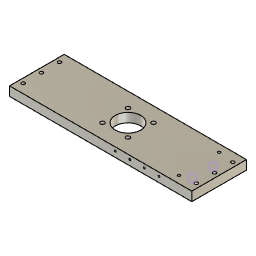
securing_structure_lid v106 (Autodesk Fusion 360 design; units mm, degrees)
Autodesk Fusion 360 part; units mm, degrees
note: some values were not read from the file. Chosen so that the rebuilt part matches the saved one: which face or edge a step refers to; how an offset face is resized; which pieces of a blend or face edit are solid. Set by a fixed rule: which sketch regions a step uses.
(part 1 of 2)
sketch "Sketch1" plane through (0, 0, 0) normal (0, 0, 1) x (1, 0, 0)
  line L0 (0, 0) -> (215, 0)
  line L1 (215, 0) -> (215, 55)
  line L2 (215, 55) -> (0, 55)
  line L3 (0, 55) -> (0, 0)
  line L4 (215, 55) -> (-215, 55)
  line L5 (-215, 55) -> (-215, -55)
  line L6 (-215, -55) -> (215, -55)
  line L7 (215, -55) -> (215, 55)
  dimension "d1" = 215
  dimension "d2" = 55
  dimension "d3" = 430
  dimension "d4" = 110
  constraint horizontal L0
  constraint vertical L1
  constraint horizontal L2
  constraint vertical L3
  constraint horizontal L4
  constraint vertical L5
  constraint horizontal L6
  constraint vertical L7
  measures "d1" distance of L0.start L0.end
  measures "d2" distance of L0.start L2.end
  measures "d3" distance of L1.end L4.end
  measures "d4" distance of L1.end L6.end
extrude "Extrude1" add sketch "Sketch1" along normal blind 170
sketch "Sketch2" plane through (0, 0, 0) normal (0, 0, 1) x (1, 0, 0)
  line L0 (0, 0) -> (-235, 0)
  line L1 (0, 0) -> (235, 0)
  line L2 (-235, 0) -> (235, 0)
  line L3 (235, 0) -> (235, 75)
  line L4 (235, 75) -> (-235, 75)
  line L5 (-235, 75) -> (-235, 0)
  line L6 (-235, 75) -> (235.5022, 75)
  line L7 (235.5022, 75) -> (235.5022, -75)
  line L8 (235.5022, -75) -> (-235, -75)
  line L9 (-235, -75) -> (-235, 75)
  line L10 (0, 0) -> (-215, 0)
  line L11 (-215, 0) -> (-215, 55)
  line L12 (-215, 55) -> (0, 55)
  line L13 (0, 55) -> (0, 0)
  line L14 (-215, 55) -> (215, 55)
  line L15 (215, 55) -> (215, -55)
  line L16 (215, -55) -> (-215, -55)
  line L17 (-215, -55) -> (-215, 55)
  dimension "d7" = 235
  dimension "d8" = 235
  dimension "d9" = 470
  dimension "d10" = 75
  dimension "d11" = 150
  dimension "d12" = 215
  dimension "d13" = 55
  dimension "d14" = 430
  dimension "d15" = 110
  constraint coincident L0.start L1.start
  constraint horizontal L0
  constraint parallel L0 L1
  constraint horizontal L2
  constraint vertical L3
  constraint horizontal L4
  constraint vertical L5
  constraint horizontal L6
  constraint vertical L7
  constraint horizontal L8
  constraint vertical L9
  constraint horizontal L10
  constraint vertical L11
  constraint horizontal L12
  constraint vertical L13
  constraint horizontal L14
  constraint vertical L15
  constraint horizontal L16
  constraint vertical L17
  measures "d7" distance of L0.start L0.end
  measures "d8" distance of L0.start L1.end
  measures "d9" distance of L0.end L1.end
  measures "d10" distance of L0.end L4.end
  measures "d11" distance of L4.end L8.end
  measures "d12" distance of L0.start L10.end
  measures "d13" distance of L0.start L12.end
  measures "d14" distance of L11.end L14.end
  measures "d15" distance of L11.end L16.end
extrude "Extrude2" add sketch "Sketch2" along normal blind 190 contours L0 L1 L2 L3 L6 L7 L8 L9 L15 L16 L17 | L0 L1 L2 L3 L4 L5 L6 L9 L11 L12 L14 L15 L17
extrude "Extrude3" add 1 faces at (-71.6667, 18.3333, 170) along direction (0, 0, 1) blind 20
sketch "Sketch3" plane through (0, 0, 0) normal (0, 0, -1) x (1, 0, 0)
  line L0 (235.5022, 75) -> (-235, 75)
  line L1 (-235, 75) -> (-235, -75)
  line L2 (-235, -75) -> (235.5022, -75)
  line L3 (235.5022, -75) -> (235.5022, 75)
  line L4 (0, 0) -> (-215, 0)
  line L5 (-215, 0) -> (-215, 55)
  line L6 (-215, 55) -> (0, 55)
  line L7 (0, 55) -> (0, 0)
  line L8 (-215, 55) -> (215, 55)
  line L9 (215, 55) -> (215, -55)
  line L10 (215, -55) -> (-215, -55)
  line L11 (-215, -55) -> (-215, 55)
  dimension "d20" = 215
  dimension "d21" = 55
  dimension "d22" = 430
  dimension "d23" = 110
  constraint horizontal L4
  constraint vertical L5
  constraint horizontal L6
  constraint vertical L7
  constraint coincident L4.start L7.end
  constraint horizontal L8
  constraint vertical L9
  constraint horizontal L10
  constraint vertical L11
  measures "d20" distance of L4.start L4.end
  measures "d21" distance of L4.start L6.end
  measures "d22" distance of L5.end L8.end
  measures "d23" distance of L5.end L10.end
extrude "Extrude4" cut sketch "Sketch3" against normal blind 170 contours L4 L7 L8 L9 L10 L11 | L4 L5 L6 L7 L8 L11
sketch "Sketch4" plane through (0, -75, 0) normal (0, -1, 0) x (1, 0, 0)
  line L0 (-235, 0) -> (235.5022, 0)
  line L1 (235.5022, 0) -> (235.5022, 190)
  line L2 (235.5022, 190) -> (-235, 190)
  line L3 (-235, 190) -> (-235, 0)
  line L4 (0, 0) -> (-215, 0)
  line L5 (-215, 0) -> (-215, 170)
  line L6 (-215, 170) -> (0, 170)
  line L7 (0, 170) -> (0, 0)
  line L8 (0, 0) -> (215, 0)
  line L9 (215, 0) -> (215, 170)
  line L10 (215, 170) -> (0, 170)
  line L11 (0, 170) -> (0, 0)
  dimension "d26" = 215
  dimension "d27" = 170
  dimension "d28" = 215
  constraint horizontal L4
  constraint vertical L5
  constraint horizontal L6
  constraint vertical L7
  constraint coincident L4.start L7.end
  constraint horizontal L8
  constraint vertical L9
  constraint horizontal L10
  constraint vertical L11
  measures "d26" distance of L4.start L4.end
  measures "d27" distance of L4.start L6.end
  measures "d28" distance of L4.start L8.end
extrude "Extrude5" cut sketch "Sketch4" against normal blind 200 contours L0 L4 L5 L6 L7 L11 | L0 L7 L8 L9 L10 L11
sketch "Sketch5" plane through (0, 0, 190) normal (0, 0, 1) x (-1, 0, 0)
  line L0 (235, 75) -> (-235.5022, 75)
  line L1 (-235.5022, 75) -> (-235.5022, -75)
  line L2 (-235.5022, -75) -> (235, -75)
  line L3 (235, -75) -> (235, 75)
  circle A0 centre (0, 0) radius 17.4
  dimension "d31" = 34.8
  constraint coincident A0.centre origin
  measures "d31" diameter of A0
extrude "Extrude6" cut sketch "Sketch5" against normal blind 60 contours A0
extrude "Extrude7" add 1 faces at (-235, 25, 63.3333) along direction (-1, 0, 0) blind 5
extrude "Extrude8" add 1 faces at (235.5022, 25, 63.3333) along direction (1, 0, 0) blind 5
extrude "Extrude9" cut 1 faces at (-215, -25, 56.6667) along direction (-1, 0, 0) blind 5
extrude "Extrude10" cut 1 faces at (215, -25, 56.6667) along direction (1, 0, 0) blind 5
extrude "Extrude11" add 1 faces at (-240, 25, 63.3333) along direction (-1, 0, 0) blind 5
extrude "Extrude12" cut 1 faces at (220, -25, 56.6667) along direction (1, 0, 0) blind 5
extrude "Extrude13" cut 1 faces at (-220, -25, 56.6667) along direction (-1, 0, 0) blind 5
extrude "Extrude14" add 1 faces at (240.5022, 25, 63.3333) along direction (1, 0, 0) blind 5
extrude "Extrude15" add 2 faces at (-231.6667, -25, 0) (238.6682, -25, 0) along direction (0, 0, -1) blind 0.719
sketch "Sketch6" plane through (-245, 0, 0) normal (-1, 0, 0) x (0, -1, 0)
  line L0 (75, -0.719) -> (75, 190)
  line L1 (75, 190) -> (-75, 190)
  line L2 (-75, 190) -> (-75, -0.719)
  line L3 (-75, -0.719) -> (75, -0.719)
  line L4 (-75, -0.719) -> (75, -0.719)
  line L5 (75, -0.719) -> (75, 19.281)
  line L6 (75, 19.281) -> (-75, 19.281)
  line L7 (-75, 19.281) -> (-75, -0.719)
  dimension "d52" = 20
  constraint horizontal L4
  constraint vertical L5
  constraint horizontal L6
  constraint vertical L7
  constraint coincident L0 L5.end
  constraint coincident L2.end L3.start
  measures "d52" distance of L2.end L6.end
extrude "Extrude16" add sketch "Sketch6" along normal blind 40 contours L0 L2 L3 L4 L5 L6 L7
sketch "Sketch7" plane through (245.5022, 0, 0) normal (1, 0, 0) x (0, 1, 0)
  line L0 (75, -0.719) -> (75, 190)
  line L1 (75, 190) -> (-75, 190)
  line L2 (-75, 190) -> (-75, -0.719)
  line L3 (-75, -0.719) -> (75, -0.719)
  line L4 (-75, -0.719) -> (75, -0.719)
  line L5 (75, -0.719) -> (75, 19.281)
  line L6 (75, 19.281) -> (-75, 19.281)
  line L7 (-75, 19.281) -> (-75, -0.719)
  dimension "d55" = 20
  constraint horizontal L4
  constraint vertical L5
  constraint horizontal L6
  constraint vertical L7
  constraint coincident L0 L5.end
  constraint coincident L2.end L3.start
  measures "d55" distance of L2.end L6.end
extrude "Extrude17" add sketch "Sketch7" along normal blind 40 contours L0 L2 L3 L4 L5 L6 L7
sketch "Sketch8" plane through (0, 0, 19.281) normal (0, 0, 1) x (-1, 0, 0)
  line L0 (-245.5022, -75) -> (-245.5022, 75)
  line L1 (-245.5022, 75) -> (-285.5022, 75)
  line L2 (-285.5022, 75) -> (-285.5022, -75)
  line L3 (-285.5022, -75) -> (-245.5022, -75)
  line L4 (-285.5022, 0) -> (-245.5022, 0)
  line L5 (-265.5022, 0) -> (-265.5022, -50)
  line L6 (-265.5022, 0) -> (-265.5022, 50)
  line L7 (-265.5022, 50) -> (264.4978, 50)
  line L8 (264.4978, 50) -> (264.4978, -50)
  line L9 (264.4978, -50) -> (-265.5022, -50)
  line L10 (-265.5022, -50) -> (-265.5022, 50)
  dimension "d58" = 50
  dimension "d59" = 50
  dimension "d60" = 530
  dimension "d61" = 100
  constraint midpoint L2 L4.start
  constraint midpoint L0 L4.end
  constraint midpoint L4 L5.start
  constraint perpendicular L3 L5
  constraint perpendicular L4 L6
  constraint horizontal L7
  constraint vertical L8
  constraint horizontal L9
  constraint vertical L10
  measures "d58" distance of L5.start L5.end
  measures "d59" distance of L5.start L6.end
  measures "d60" distance of L6.end L7.end
  measures "d61" distance of L6.end L5.end
hole "Hole1" at (265.5022, 50, 19.281) at (265.5022, -50, 19.281) at (-264.4978, -50, 19.281) at (-264.4978, 50, 19.281) direction (0, 0, -1) diameter 7.035 depth 20 tip angle 180
thread "Thread1" "ISO Metric profile 8.0 M8x1 6H"
sketch "Sketch9" plane through (0, 0, 190) normal (0, 0, 1) x (-1, 0, 0)
  circle A0 centre (0, 0) radius 17.4
  line L0 (245, 75) -> (-245.5022, 75)
  line L1 (-245.5022, 75) -> (-245.5022, -75)
  line L2 (-245.5022, -75) -> (245, -75)
  line L3 (245, -75) -> (245, 75)
  line L4 (0, 0) -> (-35, 0)
  line L5 (-35, 0) -> (-35, -35)
  line L6 (-35, -35) -> (0, -35)
  line L7 (0, -35) -> (0, 0)
  line L8 (-35, -35) -> (35, -35)
  line L9 (35, -35) -> (35, 35)
  line L10 (35, 35) -> (-35, 35)
  line L11 (-35, 35) -> (-35, -35)
  dimension "d65" = 35
  dimension "d66" = 35
  dimension "d67" = 70
  dimension "d68" = 70
  constraint horizontal L4
  constraint vertical L5
  constraint horizontal L6
  constraint vertical L7
  constraint coincident A0.centre L4.start
  constraint horizontal L8
  constraint vertical L9
  constraint horizontal L10
  constraint vertical L11
  measures "d65" distance of A0.centre L4.end
  measures "d66" distance of A0.centre L6.end
  measures "d67" distance of L5.end L8.end
  measures "d68" distance of L5.end L10.end
hole "Hole2" at (-35, 35, 190) at (35, 35, 190) at (35, -35, 190) at (-35, -35, 190) direction (0, 0, -1) diameter 7.035 depth 10 tip angle 180
thread "Thread2" "ISO Metric profile 8.0 M8x1 6H"
sketch "Sketch10" plane through (0, 0, 190) normal (0, 0, 1) x (-1, 0, 0)
  circle A0 centre (-35, 35) radius 3.5175
  circle A1 centre (35, -35) radius 3.5175
  circle A2 centre (-35, -35) radius 3.5175
  circle A3 centre (35, 35) radius 3.5175
  circle A4 centre (0, 0) radius 17.4
  line L0 (245, 75) -> (-245.5022, 75)
  line L1 (-245.5022, 75) -> (-245.5022, -75)
  line L2 (-245.5022, -75) -> (245, -75)
  line L3 (245, -75) -> (245, 75)
  circle A5 centre (0, 0) radius 15
  dimension "d72" = 30
  constraint coincident A4.centre A5.centre
  measures "d72" diameter of A5
extrude "Extrude18" add sketch "Sketch10" against normal blind 20 contours A4
delete_face "DeleteFace1" 4 faces at (35.1753, 31.4869, 186.6667) (35.1753, -38.5131, 186.6667) (-34.8247, 31.4869, 186.6667) (-34.8247, -38.5131, 186.6667)
sketch "Sketch11" plane through (0, 0, 190) normal (0, 0, 1) x (-1, 0, 0)
  circle A0 centre (0, 0) radius 15
  line L0 (245, 75) -> (-245.5022, 75)
  line L1 (-245.5022, 75) -> (-245.5022, -75)
  line L2 (-245.5022, -75) -> (245, -75)
  line L3 (245, -75) -> (245, 75)
  line L4 (0, 0) -> (35, 0)
  line L5 (35, 0) -> (35, -35)
  line L6 (35, -35) -> (0, -35)
  line L7 (0, -35) -> (0, 0)
  line L8 (35, -35) -> (-35, -35)
  line L9 (-35, -35) -> (-35, 35)
  line L10 (-35, 35) -> (35, 35)
  line L11 (35, 35) -> (35, -35)
  constraint horizontal L4
  constraint vertical L5
  constraint horizontal L6
  constraint vertical L7
  constraint coincident A0.centre L4.start
  constraint horizontal L8
  constraint vertical L9
  constraint horizontal L10
  constraint vertical L11
hole "Hole3" at (-35, 35, 190) at (35, 35, 190) at (35, -35, 190) at (-35, -35, 190) direction (0, 0, -1) diameter 6.78 depth 10 tip angle 180
thread "Thread3" "ISO Metric profile 8.0 M8x1 6H" major diameter 8.147 minor diameter 7.035 pitch 1 angle 60 resizes the face on face at (-34.831, 31.6142, 186.6667) on face at (35.169, 31.6142, 186.6667) on face at (35.169, -38.3858, 186.6667) on face at (-34.831, -38.3858, 186.6667)
extrude "Extrude19" add 1 faces at (155, 0, 170) along direction (0, 0, -1) blind 38
extrude "Extrude20" cut 1 faces at (176.4014, -11.1796, 190) along direction (0, 0, -1) blind 38
hole "Hole4" at (35, -35, 180) direction (0, 0, -1) diameter 7.035 depth 38 tip angle 180
thread "Thread4" "ISO Metric profile 8.0 M8x1 6H"
sketch "Sketch12" plane through (0, 0, 180) normal (0, 0, 1) x (-1, 0, 0)
  circle A0 centre (35, -35) radius 3.5175
hole "Hole5" at (-35, 35, 180) direction (0, 0, -1) diameter 7.035 depth 38 tip angle 180
thread "Thread5" "ISO Metric profile 8.0 M8x1 6H"
sketch "Sketch13" plane through (0, 0, 180) normal (0, 0, 1) x (-1, 0, 0)
  circle A0 centre (-35, -35) radius 3.5175
hole "Hole6" at (35, 35, 180) direction (0, 0, -1) diameter 7.035 depth 38 tip angle 180
thread "Thread6" "ISO Metric profile 8.0 M8x1 6H"
sketch "Sketch14" plane through (0, 0, 180) normal (0, 0, 1) x (-1, 0, 0)
  circle A0 centre (35, 35) radius 3.5175
hole "Hole7" at (-35, -35, 180) direction (0, 0, -1) diameter 7.035 depth 38 tip angle 180
thread "Thread7" "ISO Metric profile 8.0 M8x1 6H"
sketch "Sketch15" plane through (285.5022, 0, 0) normal (1, 0, 0) x (0, 1, 0)
  line L0 (-75, 19.281) -> (-75, -0.719)
  line L1 (-75, -0.719) -> (75, -0.719)
  line L2 (75, -0.719) -> (75, 19.281)
  line L3 (75, 19.281) -> (-75, 19.281)
  line L4 (0, -0.719) -> (0, 9.281)
  dimension "d106" = 10
  constraint midpoint L1 L4.start
  constraint perpendicular L1 L4
  measures "d106" distance of L4.start L4.end
hole "Hole8" at (285.5022, 0, 9.281) direction (-1, 0, 0) diameter 7.035 depth 20 tip angle 180
thread "Thread8" "ISO Metric profile 8.0 M8x1 6H"
delete_face "DeleteFace2" 1 faces at (-265.7008, 53.3054, 12.6143)
delete_face "DeleteFace3" 1 faces at (-265.7008, -46.6946, 12.6143)
sketch "Sketch16" plane through (0, 0, 19.281) normal (0, 0, 1) x (-1, 0, 0)
  line L0 (245, 75) -> (245, -75)
  line L1 (245, -75) -> (285, -75)
  line L2 (285, -75) -> (285, 75)
  line L3 (285, 75) -> (245, 75)
  line L4 (285, -75) -> (265, -75)
  line L5 (265, -75) -> (265, -50)
  line L6 (265, -50) -> (285, -50)
  line L7 (285, -50) -> (285, -75)
  line L8 (285, 75) -> (265, 75)
  line L9 (265, 75) -> (265, 50)
  line L10 (265, 50) -> (285, 50)
  line L11 (285, 50) -> (285, 75)
  dimension "d110" = 20
  dimension "d111" = 25
  dimension "d112" = 20
  dimension "d113" = 25
  constraint horizontal L4
  constraint vertical L5
  constraint horizontal L6
  constraint vertical L7
  constraint coincident L1.end L2.start
  constraint horizontal L8
  constraint vertical L9
  constraint horizontal L10
  constraint vertical L11
  constraint coincident L2.end L3.start
  measures "d110" distance of L1.end L4.end
  measures "d111" distance of L1.end L6.end
  measures "d112" distance of L2.end L8.end
  measures "d113" distance of L2.end L10.end
hole "Hole9" at (-265, 50, 19.281) at (-265, -50, 19.281) direction (0, 0, -1) diameter 7.035 depth 20 tip angle 180
thread "Thread9" "ISO Metric profile 8.0 M8x1 6H"
sketch "Sketch17" plane through (0, 0, 152) normal (0, 0, 1) x (-1, 0, 0)
  circle A0 centre (-35, 35) radius 3.5175
  circle A1 centre (35, -35) radius 3.5175
  circle A2 centre (-35, -35) radius 3.5175
  circle A3 centre (35, 35) radius 3.5175
  circle A4 centre (0, 0) radius 15
  line L0 (245, 75) -> (-245.5022, 75)
  line L1 (-245.5022, 75) -> (-245.5022, -75)
  line L2 (-245.5022, -75) -> (245, -75)
  line L3 (245, -75) -> (245, 75)
  line L4 (-245.5022, 0) -> (-225.5022, 0)
  dimension "d117" = 20
  constraint midpoint L1 L4.start
  constraint perpendicular L1 L4
  measures "d117" distance of L4.start L4.end
hole "Hole10" at (225.5022, 0, 152) direction (0, 0, -1) diameter 7.035 depth 10 tip angle 180
thread "Thread10" "ISO Metric profile 8.0 M8x1 6H"
extrude "Extrude21" cut 1 faces at (225, -25, 43.5207) along direction (1, 0, 0) blind 0.5
delete_face "DeleteFace4" 1 faces at (264.2992, 53.3054, 12.6143)
delete_face "DeleteFace5" 1 faces at (264.2992, -46.6946, 12.6143)
delete_face "DeleteFace6" 1 faces at (-267.6374, -52.3275, 12.6143)
delete_face "DeleteFace7" 1 faces at (-267.6374, 47.6725, 12.6143)
extrude "Extrude22" cut 1 faces at (-285, -25, 5.9477) along direction (1, 0, 0) blind 40
extrude "Extrude23" cut 1 faces at (285.5022, 51.1692, 9.3686) along direction (-1, 0, 0) blind 40
extrude "Extrude24" cut 1 faces at (265.5022, 0.8784, 8.804) along direction (-1, 0, 0) blind 20
sketch "Sketch18" plane through (0, 0, -0.719) normal (0, 0, -1) x (1, 0, 0)
  line L0 (245.5022, -75) -> (245.5022, 75)
  line L1 (245.5022, 75) -> (225.5, 75)
  line L2 (225.5, 75) -> (225.5, -75)
  line L3 (225.5, -75) -> (245.5022, -75)
  line L4 (235.5011, -75) -> (235.5011, -50)
  line L5 (235.5011, 75) -> (235.5011, 50)
  line L6 (235.5011, -50) -> (235.5011, 0)
  line L7 (-235, -75) -> (-235, -50)
  line L8 (-235, 75) -> (-235, 50)
  line L9 (-235, 50) -> (-235, 0)
  dimension "d129" = 25
  dimension "d130" = 25
  dimension "d131" = 25
  dimension "d132" = 25
  constraint midpoint L3 L4.start
  constraint perpendicular L3 L4
  constraint midpoint L1 L5.start
  constraint perpendicular L1 L5
  constraint parallel L4 L6
  constraint parallel L6 L7
  constraint vertical L8
  constraint parallel L8 L9
  measures "d129" distance of L4.start L4.end
  measures "d130" distance of L5.start L5.end
  measures "d131" distance of L7.start L7.end
  measures "d132" distance of L8.start L8.end
hole "Hole11" at (-235, -50, -0.719) at (-235, 0, -0.719) at (-235, 50, -0.719) at (235.5011, 0, -0.719) at (235.5011, -50, -0.719) at (235.5011, 50, -0.719) direction (0, 0, 1) diameter 7.035 depth 20 tip angle 180
thread "Thread11" "ISO Metric profile 8.0 M8x1 6H"
delete_face "DeleteFace8" 1 faces at (225.6776, -3.5131, 148.6667)
sketch "Sketch19" plane through (0, 0, 152) normal (0, 0, 1) x (-1, 0, 0)
  circle A0 centre (-35, 35) radius 3.5175
  circle A1 centre (35, -35) radius 3.5175
  circle A2 centre (-35, -35) radius 3.5175
  circle A3 centre (35, 35) radius 3.5175
  circle A4 centre (0, 0) radius 15
  line L0 (245, 75) -> (-245.5022, 75)
  line L1 (-245.5022, 75) -> (-245.5022, -75)
  line L2 (-245.5022, -75) -> (245, -75)
  line L3 (245, -75) -> (245, 75)
  line L4 (-245.5022, 0) -> (-245, 0)
  line L5 (-245, 0) -> (-225, 0)
  line L6 (-225, 0) -> (-225, -13.746)
  line L7 (-225, -13.746) -> (-225, 13.746)
  dimension "d136" = 20
  dimension "d137" = 13.746
  dimension "d138" = 27.492
  constraint midpoint L1 L4.start
  constraint perpendicular L1 L4
  constraint perpendicular L1 L5
  constraint perpendicular L5 L6
  constraint perpendicular L5 L7
  measures "d136" distance of L4.end L5.end
  measures "d137" distance of L5.end L6.end
  measures "d138" distance of L6.end L7.end
hole "Hole12" at (225, 13.746, 152) at (225, -13.746, 152) direction (0, 0, -1) diameter 3.529 depth 10 tip angle 180
thread "Thread12" "ISO Metric profile 4.0 M4x0.5 6H"
sketch "Sketch20" plane through (0, 0, 152) normal (0, 0, 1) x (-1, 0, 0)
  circle A0 centre (-225, -13.746) radius 1.7644
  circle A1 centre (-225, 13.746) radius 1.7644
  circle A2 centre (-35, 35) radius 3.5175
  circle A3 centre (35, -35) radius 3.5175
  circle A4 centre (-35, -35) radius 3.5175
  circle A5 centre (35, 35) radius 3.5175
  circle A6 centre (0, 0) radius 15
  line L0 (245, 75) -> (-245.5022, 75)
  line L1 (-245.5022, 75) -> (-245.5022, -75)
  line L2 (-245.5022, -75) -> (245, -75)
  line L3 (245, -75) -> (245, 75)
  line L4 (-225, -13.746) -> (-215, -13.746)
  line L5 (-215, -13.746) -> (-215, 13.746)
  dimension "d142" = 10
  constraint coincident A0.centre L4.start
  constraint horizontal L4
  constraint perpendicular L4 L5
  measures "d142" distance of A0.centre L4.end
hole "Hole13" at (215, 13.746, 152) at (215, -13.746, 152) direction (0, 0, -1) diameter 3.529 depth 10 tip angle 180
thread "Thread13" "ISO Metric profile 4.0 M4x0.5 6H"
delete_face "DeleteFace9" 1 faces at (225.9201, 15.2516, 148.6667)
delete_face "DeleteFace10" 1 faces at (225.9201, -12.2404, 148.6667)
sketch "Sketch21" plane through (245.5022, 0, 0) normal (1, 0, 0) x (0, 1, 0)
  line L0 (75, 152) -> (-75, 152)
  line L1 (-75, 152) -> (-75, -0.719)
  line L2 (-75, -0.719) -> (75, -0.719)
  line L3 (75, -0.719) -> (75, 152)
  line L4 (0, 152) -> (-28.5, 152)
  line L5 (-28.5, 152) -> (-28.5, 142)
  line L6 (-28.5, 142) -> (0, 142)
  line L7 (0, 142) -> (0, 152)
  line L8 (-28.5, 152) -> (28.5, 152)
  line L9 (28.5, 152) -> (28.5, 142)
  line L10 (28.5, 142) -> (-28.5, 142)
  line L11 (-28.5, 142) -> (-28.5, 152)
  dimension "d146" = 28.5
  dimension "d147" = 10
  dimension "d148" = 57
  dimension "d149" = 10
  constraint horizontal L4
  constraint vertical L5
  constraint horizontal L6
  constraint vertical L7
  constraint midpoint L0 L4.start
  constraint horizontal L8
  constraint vertical L9
  constraint horizontal L10
  constraint vertical L11
  measures "d146" distance of L4.start L4.end
  measures "d147" distance of L4.start L6.end
  measures "d148" distance of L4.end L8.end
  measures "d149" distance of L4.end L5.end
extrude "Extrude25" cut sketch "Sketch21" against normal blind 10 contours L0 L7 L8 L9 L10 | L0 L4 L5 L6 L7 L8 L10 L11
sketch "Sketch22" plane through (235.5022, 0, 0) normal (1, 0, 0) x (0, 1, 0)
  line L0 (-28.5, 142) -> (28.5, 142)
  line L1 (28.5, 142) -> (28.5, 152)
  line L2 (28.5, 152) -> (-28.5, 152)
  line L3 (-28.5, 152) -> (-28.5, 142)
  line L4 (0, 142) -> (0, 147)
  dimension "d152" = 5
  constraint midpoint L0 L4.start
  constraint perpendicular L0 L4
  measures "d152" distance of L4.start L4.end
hole "Hole14" at (235.5022, 0, 147) direction (-1, 0, 0) diameter 6.78 depth 10 tip angle 180
thread "Thread14" "ISO Metric profile 8.0 M8x1 6H" major diameter 8.147 minor diameter 7.035 pitch 1 angle 60 resizes the face on face at (232.1689, -3.3637, 146.5785)
extrude "Extrude26" cut 1 faces at (235.5022, -20.1692, 147.0876) along direction (-1, 0, 0) blind 10
delete_face "DeleteFace11" 1 faces at (215.9201, 15.2516, 148.6667)
delete_face "DeleteFace12" 1 faces at (215.9201, -12.2404, 148.6667)
sketch "Sketch23" plane through (0, 0, 142) normal (0, 0, 1) x (-1, 0, 0)
  line L0 (-245.5022, 28.5) -> (-245.5022, -28.5)
  line L1 (-245.5022, -28.5) -> (-225.5022, -28.5)
  line L2 (-225.5022, -28.5) -> (-225.5022, 28.5)
  line L3 (-225.5022, 28.5) -> (-245.5022, 28.5)
  line L4 (-235, 0) -> (-235, -13.746)
  line L5 (-235, 0) -> (-235, 13.746)
  line L6 (-235, -13.746) -> (-240, -13.746)
  line L7 (-240, -13.746) -> (-240, -12)
  line L8 (-240, -12) -> (-235, -12)
  line L9 (-235, -12) -> (-235, -13.746)
  line L10 (-240, -12) -> (-230, -12)
  line L11 (-230, -12) -> (-230, -13.746)
  line L12 (-230, -13.746) -> (-240, -13.746)
  line L13 (-240, -13.746) -> (-240, -12)
  line L14 (-235, 13.746) -> (-240, 13.746)
  line L15 (-240, 13.746) -> (-240, 15.492)
  line L16 (-240, 15.492) -> (-235, 15.492)
  line L17 (-235, 15.492) -> (-235, 13.746)
  line L18 (-230, -12) -> (-240, -12)
  line L19 (-240, -12) -> (-240, -10.254)
  line L20 (-240, -10.254) -> (-230, -10.254)
  line L21 (-230, -10.254) -> (-230, -12)
  line L22 (-240, 13.746) -> (-230, 13.746)
  line L23 (-230, 13.746) -> (-230, 12)
  line L24 (-230, 12) -> (-240, 12)
  line L25 (-240, 12) -> (-240, 13.746)
  line L26 (-240, 12) -> (-230, 12)
  line L27 (-230, 12) -> (-230, 15.492)
  line L28 (-230, 15.492) -> (-240, 15.492)
  line L29 (-240, 15.492) -> (-240, 12)
  dimension "d158" = 13.746
  dimension "d159" = 13.746
  dimension "d160" = 5
  dimension "d161" = 1.746
  dimension "d162" = 10
  dimension "d163" = 5
  dimension "d164" = 1.746
  dimension "d165" = 10
  dimension "d166" = 1.746
  dimension "d167" = 10
  dimension "d168" = 1.746
  dimension "d169" = 3.492
  constraint vertical L4
  constraint parallel L2 L5
  constraint horizontal L6
  constraint vertical L7
  constraint horizontal L8
  constraint vertical L9
  constraint horizontal L10
  constraint vertical L11
  constraint horizontal L12
  constraint vertical L13
  constraint horizontal L14
  constraint vertical L15
  constraint horizontal L16
  constraint vertical L17
  constraint horizontal L18
  constraint vertical L19
  constraint horizontal L20
  constraint vertical L21
  constraint horizontal L22
  constraint vertical L23
  constraint horizontal L24
  constraint vertical L25
  constraint horizontal L26
  constraint vertical L27
  constraint horizontal L28
  constraint vertical L29
  measures "d158" distance of L4.start L4.end
  measures "d159" distance of L4.start L5.end
  measures "d160" distance of L4.end L6.end
  measures "d161" distance of L4.end L8.end
  measures "d162" distance of L7.end L10.end
  measures "d163" distance of L5.end L14.end
  measures "d164" distance of L5.end L16.end
  measures "d165" distance of L10.end L7.end
  measures "d166" distance of L10.end L20.end
  measures "d167" distance of L14.end L22.end
  measures "d168" distance of L14.end L24.end
  measures "d169" distance of L24.end L15.end
extrude "Extrude27" cut sketch "Sketch23" against normal blind 2 contours L4 L9 L10 L11 L12 L18 | L4 L8 L10 L18 L19 L20 | L4 L6 L7 L8 L9 L10 L12 L13 L18 | L4 L10 L18 L20 L21 | L5 L14 L22 L24 L25 L26 L29 | L5 L22 L23 L24 L26 L27 | L14 L15 L16 L17 L22 L28 L29 | L17 L22 L27 L28
extrude "Extrude28" cut 1 faces at (225.5022, -9.5, 145.3333) along direction (-1, 0, 0) blind 20.502
extrude "Extrude29" cut 2 faces at (230, -14.328, 141.3333) (230, -13.164, 141.3333) along direction (-1, 0, 0) blind 20
extrude "Extrude30" cut 1 faces at (230, 11.418, 141.3333) along direction (-1, 0, 0) blind 20
sketch "Sketch24" plane through (205.0002, 0, 0) normal (1, 0, 0) x (0, 1, 0)
  line L0 (-28.5, 142) -> (28.5, 142)
  line L1 (28.5, 142) -> (28.5, 152)
  line L2 (28.5, 152) -> (-28.5, 152)
  line L3 (-28.5, 152) -> (-28.5, 142)
  line L4 (0, 142) -> (0, 147)
  dimension "d178" = 5
  constraint midpoint L0 L4.start
  constraint perpendicular L0 L4
  measures "d178" distance of L4.start L4.end
hole "Hole15" at (205.0002, 0, 147) direction (-1, 0, 0) diameter 7.035 depth 10 tip angle 180
thread "Thread15" "ISO Metric profile 8.0 M8x1 6H"
sketch "Sketch25" plane through (0, 0, 142) normal (0, 0, 1) x (-1, 0, 0)
  line L0 (-210, -13.746) -> (-240, -13.746)
  line L1 (-240, -13.746) -> (-240, -10.254)
  line L2 (-240, -10.254) -> (-210, -10.254)
  line L3 (-210, -10.254) -> (-210, -13.746)
  line L4 (-210, 12) -> (-240, 12)
  line L5 (-240, 12) -> (-240, 15.492)
  line L6 (-240, 15.492) -> (-210, 15.492)
  line L7 (-210, 15.492) -> (-210, 12)
  line L8 (-245.5022, 28.5) -> (-245.5022, -28.5)
  line L9 (-245.5022, -28.5) -> (-205.0002, -28.5)
  line L10 (-205.0002, 28.5) -> (-245.5022, 28.5)
extrude "Extrude31" add 1 faces at (210, 11.418, 141.3333) along direction (1, 0, 0) blind 5
extrude "Extrude32" add 2 faces at (210, -13.164, 141.3333) (210, -14.328, 141.3333) along direction (1, 0, 0) blind 5
extrude "Extrude33" add 1 faces at (215, 11.418, 141.3333) along direction (1, 0, 0) blind 25
extrude "Extrude34" add 2 faces at (215, -13.164, 141.3333) (215, -14.328, 141.3333) along direction (1, 0, 0) blind 25
delete_face "DeleteFace13" 1 faces at (201.6669, 2.261, 149.6946)
extrude "Extrude35" add 1 faces at (205.0002, -9.5, 145.3333) along direction (1, 0, 0) blind 0.502
sketch "Sketch26" plane through (205.5022, 0, 0) normal (1, 0, 0) x (0, 1, 0)
  line L0 (-28.5, 142) -> (28.5, 142)
  line L1 (28.5, 142) -> (28.5, 152)
  line L2 (28.5, 152) -> (-28.5, 152)
  line L3 (-28.5, 152) -> (-28.5, 142)
  line L4 (0, 142) -> (0, 147)
  dimension "d193" = 5
  constraint midpoint L0 L4.start
  constraint perpendicular L0 L4
  measures "d193" distance of L4.start L4.end
hole "Hole16" at (205.5022, 0, 147) direction (-1, 0, 0) diameter 6.78 depth 20 tip angle 180
thread "Thread16" "ISO Metric profile 8.0 M8x1 6H" major diameter 8.147 minor diameter 7.035 pitch 1 angle 60 resizes the face on face at (198.8356, -3.3637, 146.5785)
delete_face "DeleteFace14" 1 faces at (235.8513, -46.5, 12.6143)
delete_face "DeleteFace15" 1 faces at (235.8513, 3.5, 12.6143)
delete_face "DeleteFace16" 1 faces at (235.8513, 53.5, 12.6143)
extrude "Extrude36" cut 1 faces at (232.1674, -25, -0.719) along direction (0, 0, 1) blind 132.719
delete_face "DeleteFace17" 2 faces at (-234.6498, 3.5, 12.6143) (-235.8492, 0.692, 19.281)
delete_face "DeleteFace18" 2 faces at (-234.6498, -46.5, 12.6143) (-236.1692, -51.0849, 19.281)
delete_face "DeleteFace19" 1 faces at (-234.6498, 53.5, 12.6143)
extrude "Extrude37" cut 1 faces at (-231.6667, 25, -0.719) along direction (0, 0, 1) blind 132.719
sketch "Sketch27" plane through (0, 0, 152) normal (0, 0, 1) x (-1, 0, 0)
  line L0 (-245.5022, 28.5) -> (-205.5022, 28.5)
  line L1 (-205.5022, 28.5) -> (-205.5022, -28.5)
  line L2 (-205.5022, -28.5) -> (-245.5022, -28.5)
  line L3 (-245.5022, -28.5) -> (-245.5022, -75)
  line L4 (-245.5022, -75) -> (245, -75)
  line L5 (245, -75) -> (245, 75)
  line L6 (245, 75) -> (-245.5022, 75)
  line L7 (-245.5022, 75) -> (-245.5022, 28.5)
  circle A0 centre (0, 0) radius 15
  circle A1 centre (35, 35) radius 3.5175
  circle A2 centre (-35, -35) radius 3.5175
  circle A3 centre (35, -35) radius 3.5175
  circle A4 centre (-35, 35) radius 3.5175
  line L8 (245, -75) -> (235, -75)
  line L9 (235, -75) -> (235, -50)
  line L10 (245, 75) -> (235, 75)
  line L11 (235, 75) -> (235, 50)
  line L12 (-245.5022, -75) -> (-235.5022, -75)
  line L13 (-245.5022, 75) -> (-235.5022, 75)
  line L14 (-235.5022, 75) -> (-235.5022, 50)
  line L15 (-235.5022, -75) -> (-235.5022, -50)
  dimension "d201" = 10
  dimension "d202" = 25
  dimension "d203" = 10
  dimension "d204" = 25
  dimension "d206" = 10
  dimension "d207" = 25
  dimension "d208" = 25
  constraint coincident L4.end L5.start
  constraint perpendicular L5 L8
  constraint perpendicular L8 L9
  constraint coincident L5.end L6.start
  constraint perpendicular L5 L10
  constraint perpendicular L10 L11
  constraint coincident L3.end L4.start
  constraint perpendicular L3 L12
  constraint coincident L6.end L7.start
  constraint perpendicular L7 L13
  constraint perpendicular L13 L14
  constraint perpendicular L12 L15
  measures "d201" distance of L4.end L8.end
  measures "d202" distance of L8.end L9.end
  measures "d203" distance of L5.end L10.end
  measures "d204" distance of L10.end L11.end
  measures "d206" distance of L6.end L13.end
  measures "d207" distance of L13.end L14.end
  measures "d208" distance of L12.end L15.end
hole "Hole17" at (-235, 50, 152) at (-235, -50, 152) at (235.5022, 50, 152) at (235.5022, -50, 152) direction (0, 0, -1) diameter 6.78 depth 60 tip angle 180
sketch "Sketch28" plane through (0, 0, 132) normal (0, 0, 1) x (-1, 0, 0)
  circle A0 centre (235, -50) radius 3.5175
  circle A1 centre (235, 50) radius 3.5175
  line L0 (245, -75) -> (245, 75)
  line L1 (245, 75) -> (225, 75)
  line L2 (225, 75) -> (225, -75)
  line L3 (225, -75) -> (245, -75)
  line L4 (235, -50) -> (235, 0)
  constraint coincident A0.centre L4.start
  constraint vertical L4
sketch "Sketch29" plane through (0, 0, 152) normal (0, 0, 1) x (-1, 0, 0)
  circle A0 centre (-235.5022, -50) radius 3.39
  circle A1 centre (235, -50) radius 3.39
  circle A2 centre (235, 50) radius 3.39
  circle A3 centre (-235.5022, 50) radius 3.39
  line L0 (-245.5022, 28.5) -> (-205.5022, 28.5)
  line L1 (-205.5022, 28.5) -> (-205.5022, -28.5)
  line L2 (-205.5022, -28.5) -> (-245.5022, -28.5)
  line L3 (-245.5022, -28.5) -> (-245.5022, -75)
  line L4 (-245.5022, -75) -> (245, -75)
  line L5 (245, -75) -> (245, 75)
  line L6 (245, 75) -> (-245.5022, 75)
  line L7 (-245.5022, 75) -> (-245.5022, 28.5)
  circle A4 centre (0, 0) radius 15
  circle A5 centre (35, 35) radius 3.5175
  circle A6 centre (-35, -35) radius 3.5175
  circle A7 centre (35, -35) radius 3.5175
  circle A8 centre (-35, 35) radius 3.5175
  line L8 (235, -50) -> (235, 0)
  constraint coincident A1.centre L8.start
  constraint vertical L8
hole "Hole18" at (-235, 0, 152) direction (0, 0, -1) diameter 6.78 depth 80 tip angle 180
delete_face "DeleteFace20" 1 faces at (192.1689, -2.856, 144.9467)
move_face "OffsetFaces1" offset 10 1 faces at (218.8356, -9.5, 142)
sketch "Sketch30" plane through (0, 0, 152) normal (0, 0, 1) x (-1, 0, 0)
  circle A0 centre (-35, 35) radius 3.5175
  circle A1 centre (35, -35) radius 3.5175
  circle A2 centre (-35, -35) radius 3.5175
  circle A3 centre (35, 35) radius 3.5175
  circle A4 centre (0, 0) radius 15
  circle A5 centre (-235.5022, 50) radius 3.39
  circle A6 centre (235, 50) radius 3.39
  circle A7 centre (235, -50) radius 3.39
  circle A8 centre (-235.5022, -50) radius 3.39
  circle A9 centre (235, 0) radius 3.39
  line L0 (-245.5022, 75) -> (-245.5022, -75)
  line L1 (-245.5022, -75) -> (245, -75)
  line L2 (245, -75) -> (245, 75)
  line L3 (245, 75) -> (-245.5022, 75)
  line L4 (-245.5022, 0) -> (-235.5022, 0)
  line L5 (-235.5022, 0) -> (-235.5022, -13.746)
  line L6 (-235.5022, -13.746) -> (-245.5022, -13.746)
  line L7 (-245.5022, -13.746) -> (-245.5022, 0)
  line L8 (-235.5022, 0) -> (-235.5022, 13.746)
  dimension "d246" = 10
  dimension "d247" = 13.746
  dimension "d248" = 13.746
  constraint horizontal L4
  constraint vertical L5
  constraint horizontal L6
  constraint vertical L7
  constraint midpoint L0 L4.start
  constraint perpendicular L4 L8
  measures "d246" distance of L4.start L4.end
  measures "d247" distance of L4.start L6.end
  measures "d248" distance of L4.end L8.end
hole "Hole19" at (235.5022, 13.746, 152) at (235.5022, -13.746, 152) direction (0, 0, -1) diameter 6.6 depth 50 tip angle 180
sketch "Sketch31" plane through (0, 0, 152) normal (0, 0, 1) x (-1, 0, 0)
  circle A0 centre (-235.5022, -13.746) radius 3.3
  circle A1 centre (-235.5022, 13.746) radius 3.3
  circle A2 centre (-35, 35) radius 3.5175
  circle A3 centre (35, -35) radius 3.5175
  circle A4 centre (-35, -35) radius 3.5175
  circle A5 centre (35, 35) radius 3.5175
  circle A6 centre (0, 0) radius 15
  circle A7 centre (-235.5022, 50) radius 3.39
  circle A8 centre (235, 50) radius 3.39
  circle A9 centre (235, -50) radius 3.39
  circle A10 centre (-235.5022, -50) radius 3.39
  circle A11 centre (235, 0) radius 3.39
  line L0 (-245.5022, 75) -> (-245.5022, -75)
  line L1 (-245.5022, -75) -> (245, -75)
  line L2 (245, -75) -> (245, 75)
  line L3 (245, 75) -> (-245.5022, 75)
  circle A12 centre (0, 0) radius 19
  dimension "d252" = 38
  constraint coincident A6.centre A12.centre
  measures "d252" diameter of A12
extrude "Extrude38" cut sketch "Sketch31" against normal blind 70 contours A12
sketch "Sketch32" plane through (0, 0, 152) normal (0, 0, 1) x (-1, 0, 0)
  circle A0 centre (0, 0) radius 19
  circle A1 centre (-235.5022, -13.746) radius 3.3
  circle A2 centre (-235.5022, 13.746) radius 3.3
  circle A3 centre (-35, 35) radius 3.5175
  circle A4 centre (35, -35) radius 3.5175
  circle A5 centre (-35, -35) radius 3.5175
  circle A6 centre (35, 35) radius 3.5175
  circle A7 centre (-235.5022, 50) radius 3.39
  circle A8 centre (235, 50) radius 3.39
  circle A9 centre (235, -50) radius 3.39
  circle A10 centre (-235.5022, -50) radius 3.39
  circle A11 centre (235, 0) radius 3.39
  line L0 (-245.5022, 75) -> (-245.5022, -75)
  line L1 (-245.5022, -75) -> (245, -75)
  line L2 (245, -75) -> (245, 75)
  line L3 (245, 75) -> (-245.5022, 75)
  circle A12 centre (0, 0) radius 20
  dimension "d255" = 40
  constraint coincident A0.centre A12.centre
  measures "d255" diameter of A12
extrude "Extrude39" cut sketch "Sketch32" against normal blind 35 contours A12
delete_face "DeleteFace21" 1 faces at (-19.9006, 1.9914, 145.3333)
sketch "Sketch33" plane through (0, 0, 152) normal (0, 0, 1) x (-1, 0, 0)
  circle A0 centre (-235.5022, -13.746) radius 3.3
  circle A1 centre (-235.5022, 13.746) radius 3.3
  circle A2 centre (-35, 35) radius 3.5175
  circle A3 centre (35, -35) radius 3.5175
  circle A4 centre (-35, -35) radius 3.5175
  circle A5 centre (35, 35) radius 3.5175
  circle A6 centre (-235.5022, 50) radius 3.39
  circle A7 centre (235, 50) radius 3.39
  circle A8 centre (235, -50) radius 3.39
  circle A9 centre (-235.5022, -50) radius 3.39
  circle A10 centre (235, 0) radius 3.39
  line L0 (-245.5022, 75) -> (-245.5022, -75)
  line L1 (-245.5022, -75) -> (245, -75)
  line L2 (245, -75) -> (245, 75)
  line L3 (245, 75) -> (-245.5022, 75)
  line L4 (245, -75) -> (-0.251, -75)
  line L5 (-0.251, -75) -> (-0.2511, 75)
  line L6 (-0.2511, 75) -> (-0.2511, 0)
  circle A11 centre (-0.2511, 0) radius 20
  dimension "d258" = 245.251
  dimension "d259" = 150
  dimension "d260" = 75
  dimension "d261" = 40
  constraint coincident L1.end L2.start
  constraint perpendicular L0 L4
  constraint midpoint L3 L5.end
  constraint perpendicular L3 L6
  constraint coincident L6.end A11.centre
  measures "d258" distance of L1.end L4.end
  measures "d259" distance of L4.end L5.end
  measures "d260" distance of L5.end L6.end
  measures "d261" diameter of A11
extrude "Extrude40" cut sketch "Sketch33" against normal blind 25 contours L5 L6 A11 | L5 L6 A11
delete_face "DeleteFace22" 1 faces at (35.3502, -38.5, 145.3333)
delete_face "DeleteFace23" 1 faces at (-34.6498, -38.5, 145.3333)
delete_face "DeleteFace24" 1 faces at (-34.6498, 31.5, 145.3333)
delete_face "DeleteFace25" 1 faces at (35.3502, 31.5, 145.3333)
sketch "Sketch34" plane through (0, 0, 152) normal (0, 0, 1) x (-1, 0, 0)
  circle A0 centre (-0.2511, 0) radius 20
  circle A1 centre (-235.5022, -13.746) radius 3.3
  circle A2 centre (-235.5022, 13.746) radius 3.3
  circle A3 centre (-235.5022, 50) radius 3.39
  circle A4 centre (235, 50) radius 3.39
  circle A5 centre (235, -50) radius 3.39
  circle A6 centre (-235.5022, -50) radius 3.39
  circle A7 centre (235, 0) radius 3.39
  line L0 (-245.5022, 75) -> (-245.5022, -75)
  line L1 (-245.5022, -75) -> (245, -75)
  line L2 (245, -75) -> (245, 75)
  line L3 (245, 75) -> (-245.5022, 75)
  line L4 (0, 0) -> (-35, 0)
  line L5 (-35, 0) -> (-35, -35)
  line L6 (-35, -35) -> (0, -35)
  line L7 (0, -35) -> (0, 0)
  line L8 (-35, -35) -> (35, -35)
  line L9 (35, -35) -> (35, 35)
  line L10 (35, 35) -> (-35, 35)
  line L11 (-35, 35) -> (-35, -35)
  dimension "d264" = 35
  dimension "d265" = 35
  dimension "d266" = 70
  dimension "d267" = 70
  constraint horizontal L4
  constraint vertical L5
  constraint horizontal L6
  constraint vertical L7
  constraint coincident L4.start L7.end
  constraint horizontal L8
  constraint vertical L9
  constraint horizontal L10
  constraint vertical L11
  measures "d264" distance of L4.start L4.end
  measures "d265" distance of L4.start L6.end
  measures "d266" distance of L5.end L8.end
  measures "d267" distance of L5.end L10.end
hole "Hole20" at (-35, 35, 152) at (-35, -35, 152) at (35, -35, 152) at (35, 35, 152) direction (0, 0, -1) diameter 8.526 depth 5 tip angle 180
thread "Thread19" "ISO Metric profile 10.0 M10x1 6H" major diameter 10.1472 minor diameter 9.0355 pitch 1 angle 60 resizes the face on face at (-34.7875, 30.7423, 150.3333) on face at (-34.7875, -39.2577, 150.3333) on face at (35.2125, -39.2577, 150.3333) on face at (35.2125, 30.7423, 150.3333)
delete_face "DeleteFace26" 1 faces at (-19.724, 0.9969, 138.6667)
sketch "Sketch35" plane through (0, 0, 152) normal (0, 0, 1) x (-1, 0, 0)
  circle A0 centre (-35, 35) radius 4.5178
  circle A1 centre (35, -35) radius 4.5178
  circle A2 centre (35, 35) radius 4.5178
  circle A3 centre (-35, -35) radius 4.5178
  circle A4 centre (-235.5022, -13.746) radius 3.3
  circle A5 centre (-235.5022, 13.746) radius 3.3
  circle A6 centre (-235.5022, 50) radius 3.39
  circle A7 centre (235, 50) radius 3.39
  circle A8 centre (235, -50) radius 3.39
  circle A9 centre (-235.5022, -50) radius 3.39
  circle A10 centre (235, 0) radius 3.39
  line L0 (-245.5022, 75) -> (-245.5022, -75)
  line L1 (-245.5022, -75) -> (245, -75)
  line L2 (245, -75) -> (245, 75)
  line L3 (245, 75) -> (-245.5022, 75)
  circle A11 centre (0, 0) radius 18
  dimension "d271" = 36
  constraint coincident A11.centre origin
  measures "d271" diameter of A11
extrude "Extrude41" cut sketch "Sketch35" against normal blind 20 contours A11
sketch "Sketch36" plane through (0, 0, 152) normal (0, 0, 1) x (-1, 0, 0)
  circle A0 centre (0, 0) radius 18
  circle A1 centre (-35, 35) radius 4.5178
  circle A2 centre (35, -35) radius 4.5178
  circle A3 centre (35, 35) radius 4.5178
  circle A4 centre (-35, -35) radius 4.5178
  circle A5 centre (-235.5022, -13.746) radius 3.3
  circle A6 centre (-235.5022, 13.746) radius 3.3
  circle A7 centre (-235.5022, 50) radius 3.39
  circle A8 centre (235, 50) radius 3.39
  circle A9 centre (235, -50) radius 3.39
  circle A10 centre (-235.5022, -50) radius 3.39
  circle A11 centre (235, 0) radius 3.39
  line L0 (-245.5022, 75) -> (-245.5022, -75)
  line L1 (-245.5022, -75) -> (245, -75)
  line L2 (245, -75) -> (245, 75)
  line L3 (245, 75) -> (-245.5022, 75)
  circle A12 centre (0, 0) radius 23
  dimension "d274" = 46
  constraint concentric A0 A12
  measures "d274" diameter of A12
extrude "Extrude42" cut sketch "Sketch36" against normal blind 20 contours A12
sketch "Sketch37" plane through (0, 0, 152) normal (0, 0, 1) x (-1, 0, 0)
  circle A0 centre (0, 0) radius 23
  circle A1 centre (-35, 35) radius 4.5178
  circle A2 centre (35, -35) radius 4.5178
  circle A3 centre (35, 35) radius 4.5178
  circle A4 centre (-35, -35) radius 4.5178
  circle A5 centre (-235.5022, -13.746) radius 3.3
  circle A6 centre (-235.5022, 13.746) radius 3.3
  circle A7 centre (-235.5022, 50) radius 3.39
  circle A8 centre (235, 50) radius 3.39
  circle A9 centre (235, -50) radius 3.39
  circle A10 centre (-235.5022, -50) radius 3.39
  circle A11 centre (235, 0) radius 3.39
  line L0 (-245.5022, 75) -> (-245.5022, -75)
  line L1 (-245.5022, -75) -> (245, -75)
  line L2 (245, -75) -> (245, 75)
  line L3 (245, 75) -> (-245.5022, 75)
  circle A12 centre (0, 0) radius 35
  dimension "d277" = 70
  constraint concentric A0 A12
  measures "d277" diameter of A12
extrude "Extrude43" cut sketch "Sketch37" against normal blind 30 contours A12
sketch "Sketch38" plane through (0, 0, 152) normal (0, 0, 1) x (-1, 0, 0)
  circle A0 centre (0, 0) radius 35
  circle A1 centre (-35, 35) radius 4.5178
  circle A2 centre (35, -35) radius 4.5178
  circle A3 centre (35, 35) radius 4.5178
  circle A4 centre (-35, -35) radius 4.5178
  circle A5 centre (-235.5022, -13.746) radius 3.3
  circle A6 centre (-235.5022, 13.746) radius 3.3
  circle A7 centre (-235.5022, 50) radius 3.39
  circle A8 centre (235, 50) radius 3.39
  circle A9 centre (235, -50) radius 3.39
  circle A10 centre (-235.5022, -50) radius 3.39
  circle A11 centre (235, 0) radius 3.39
  line L0 (-245.5022, 75) -> (-245.5022, -75)
  line L1 (-245.5022, -75) -> (245, -75)
  line L2 (245, -75) -> (245, 75)
  line L3 (245, 75) -> (-245.5022, 75)
  circle A12 centre (0, 0) radius 37.5
  dimension "d280" = 75
  constraint coincident A0.centre A12.centre
  measures "d280" diameter of A12
extrude "Extrude44" cut sketch "Sketch38" against normal blind 24 contours A12
delete_face "DeleteFace27" 1 faces at (233.924, -16.6441, 138.6667)
delete_face "DeleteFace28" 1 faces at (233.924, 10.8479, 138.6667)
sketch "Sketch39" plane through (0, 0, 152) normal (0, 0, 1) x (-1, 0, 0)
  circle A0 centre (0, 0) radius 37.5
  circle A1 centre (-35, 35) radius 4.5178
  circle A2 centre (35, -35) radius 4.5178
  circle A3 centre (35, 35) radius 4.5178
  circle A4 centre (-35, -35) radius 4.5178
  circle A5 centre (-235.5022, 50) radius 3.39
  circle A6 centre (235, 50) radius 3.39
  circle A7 centre (235, -50) radius 3.39
  circle A8 centre (-235.5022, -50) radius 3.39
  circle A9 centre (235, 0) radius 3.39
  line L0 (-245.5022, 75) -> (-245.5022, -75)
  line L1 (-245.5022, -75) -> (245, -75)
  line L2 (245, -75) -> (245, 75)
  line L3 (245, 75) -> (-245.5022, 75)
  line L4 (-235.5022, 50) -> (-235.5022, 0)
  constraint coincident A5.centre L4.start
  constraint vertical L4
hole "Hole21" at (235.5022, 0, 152) direction (0, 0, -1) diameter 6.6 depth 49 tip angle 180
sketch "Sketch40" plane through (0, 0, 152) normal (0, 0, 1) x (-1, 0, 0)
  circle A0 centre (-235.5022, 0) radius 3.3
  circle A1 centre (0, 0) radius 37.5
  circle A2 centre (-35, 35) radius 4.5178
  circle A3 centre (35, -35) radius 4.5178
  circle A4 centre (35, 35) radius 4.5178
  circle A5 centre (-35, -35) radius 4.5178
  circle A6 centre (-235.5022, 50) radius 3.39
  circle A7 centre (235, 50) radius 3.39
  circle A8 centre (235, -50) radius 3.39
  circle A9 centre (-235.5022, -50) radius 3.39
  circle A10 centre (235, 0) radius 3.39
  line L0 (-245.5022, 75) -> (-245.5022, -75)
  line L1 (-245.5022, -75) -> (245, -75)
  line L2 (245, -75) -> (245, 75)
  line L3 (245, 75) -> (-245.5022, 75)
  line L4 (-245.5022, 0) -> (-245.5022, -28.5)
  line L5 (-245.5022, -28.5) -> (-219.2482, -28.5)
  line L6 (-219.2482, -28.5) -> (-219.2482, -13.746)
  line L7 (-219.2482, -13.746) -> (-245.5022, -13.746)
  line L8 (-245.5022, -13.746) -> (-245.5022, -28.5)
  line L9 (-219.2482, -13.746) -> (-191.7562, -13.746)
  line L10 (-191.7562, -13.746) -> (-191.7562, 13.746)
  line L11 (-191.7562, 13.746) -> (-219.2482, 13.746)
  line L12 (-219.2482, 13.746) -> (-219.2482, -13.746)
  dimension "d286" = 28.5
  dimension "d287" = 26.254
  dimension "d288" = 14.754
  dimension "d289" = 27.492
  dimension "d290" = 27.492
  constraint midpoint L0 L4.start
  constraint parallel L0 L4
  constraint horizontal L5
  constraint vertical L6
  constraint horizontal L7
  constraint vertical L8
  constraint horizontal L9
  constraint vertical L10
  constraint horizontal L11
  constraint vertical L12
  measures "d286" distance of L4.start L4.end
  measures "d287" distance of L4.end L5.end
  measures "d288" distance of L4.end L7.end
  measures "d289" distance of L6.end L9.end
  measures "d290" distance of L6.end L11.end
extrude "Extrude45" add 1 faces at (167.2362, -18.6801, 132) along direction (0, 0, -1) blind 5
extrude "Extrude46" add 1 faces at (245.5022, -25, 135.3333) along direction (1, 0, 0) blind 5.25
extrude "Extrude47" add 1 faces at (-245, -25, 143.6667) along direction (-1, 0, 0) blind 5.25
delete_face "DeleteFace29" 1 faces at (-236.1594, -46.8144, 135.3333)
delete_face "DeleteFace30" 1 faces at (-234.3283, -3.3228, 135.3333)
delete_face "DeleteFace31" 1 faces at (-236.1594, 53.1856, 135.3333)
delete_face "DeleteFace32" 1 faces at (234.3428, 53.1856, 135.3333)
delete_face "DeleteFace33" 1 faces at (235.6667, -3.2959, 135.3333)
delete_face "DeleteFace34" 1 faces at (236.3387, -46.7148, 135.3333)